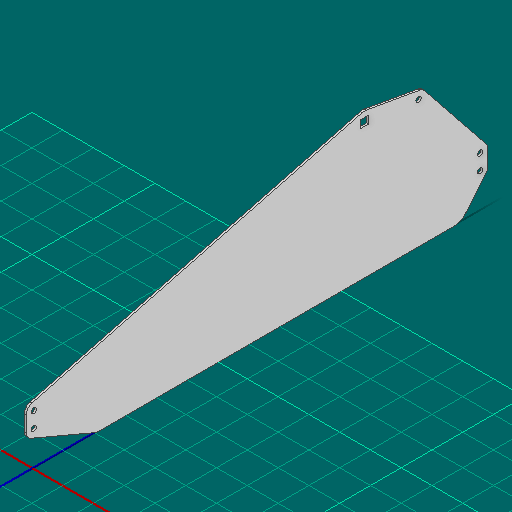
# Autodesk Inventor part: skirt_updated
Saved by Autodesk Inventor 2025 (Build 290162000, 162)
## iProperties
Created: 2024-09-29
Part Number: skirt_updated
Material: Generic
Document SubType Name: Modeling
Designer: averey
Density: 1 g/cm^3
Appearance: Default
Author: averey
Autodesk Inventor part; units mm, degrees
ref_plane "YZ Plane" through (0, 0, 0) normal (1, 0, 0) x (0, 1, 0)
ref_plane "XZ Plane" through (0, 0, 0) normal (0, 1, 0) x (-1, 0, 0)
ref_plane "XY Plane" through (0, 0, 0) normal (0, 0, 1) x (1, 0, 0)
sketch "maiin" plane through (0, 0, 0) normal (0, 0, 1) x (1, 0, 0)
  circle A0 centre (114.3234, 350.4213) radius 2.1844
  circle A1 centre (127.0234, 350.4213) radius 2.1844
  line L0 (86.4201, 300.7833) -> (108.4755, 352.8962)
  arc A2 (86.4201, 300.7833) -> (85.4157, 295.8335) centre (98.1157, 295.8335) ccw
  line L1 (209.5734, 102.7713) -> (133.0946, 352.2822)
  line L2 (209.5734, 96.4213) -> (209.5734, 102.7713)
  circle A3 centre (203.2234, 96.4213) radius 2.1844
  arc A4 (209.45, 95.176) -> (209.5734, 96.4213) centre (203.2234, 96.4213) ccw
  line L3 (196.75, 31.676) -> (209.45, 95.176)
  circle A5 centre (190.5234, 32.9213) radius 2.1844
  line L4 (85.4157, 295.8335) -> (85.4157, 3.6912)
  circle A6 centre (127.0234, -17.8787) radius 2.1844
  circle A7 centre (114.3234, -17.8787) radius 2.1844
  arc A8 (127.0234, -24.2287) -> (130.9902, -22.8372) centre (127.0234, -17.8787) ccw
  arc A9 (110.2871, -22.7809) -> (114.3234, -24.2287) centre (114.3234, -17.8787) ccw
  arc A10 (194.4902, 27.9628) -> (196.75, 31.676) centre (190.5234, 32.9213) ccw
  arc A11 (85.4157, 3.6912) -> (90.0433, -6.1132) centre (98.1157, 3.6912) ccw
  line L5 (130.9902, -22.8372) -> (194.4902, 27.9628)
  line L6 (110.2871, -22.7809) -> (90.0433, -6.1132)
  line L7 (114.3234, -24.2287) -> (127.0234, -24.2287)
  arc A12 (114.3234, 356.7713) -> (108.4755, 352.8962) centre (114.3234, 350.4213) ccw
  line L8 (127.0234, 356.7713) -> (114.3234, 356.7713)
  arc A13 (133.0946, 352.2822) -> (127.0234, 356.7713) centre (127.0234, 350.4213) ccw
  point P0 (137.6055, 139.9011)
  point P1 (110.8157, 355.7146)
  dimension "d0" = 12.7
  dimension "d1" = 12.7
  dimension "d2" = 25.4
  measures "d0" diameter of A4
  measures "d1" radius of A11
  measures "d2" distance from line of point (110.816, 355.715) L4
sketch "main" plane through (0, 0, 0) normal (0, 0, 1) x (1, 0, 0)
  line L0 (253.2515, -237.7425) -> (261.0416, -193.5682)
  circle A0 centre (170.798, 80.8603) radius 2.1844
  circle A1 centre (183.498, 80.8603) radius 2.1844
  circle A2 centre (246.998, -236.6397) radius 2.1844
  arc A3 (189.6416, 82.4661) -> (183.498, 87.2103) centre (183.498, 80.8603) ccw
  arc A4 (170.798, 87.2103) -> (164.9502, 83.3353) centre (170.798, 80.8603) ccw
  line L1 (183.498, 87.2103) -> (170.798, 87.2103)
  line L2 (141.8904, 26.2725) -> (141.8904, -265.8697)
  line L3 (260.9042, -190.1825) -> (189.6416, 82.4661)
  arc A5 (142.8948, 31.2224) -> (141.8904, 26.2725) centre (154.5904, 26.2725) ccw
  line L4 (142.8948, 31.2224) -> (164.9502, 83.3353)
  arc A6 (250.9648, -241.5982) -> (253.2515, -237.7425) centre (246.998, -236.6397) ccw
  line L5 (187.4648, -292.3982) -> (250.9648, -241.5982)
  circle A7 centre (183.498, -287.4397) radius 2.1844
  arc A8 (183.498, -293.7897) -> (187.4648, -292.3982) centre (183.498, -287.4397) ccw
  circle A9 centre (170.798, -287.4397) radius 2.1844
  line L6 (170.798, -293.7897) -> (183.498, -293.7897)
  arc A10 (166.7618, -292.3419) -> (170.798, -293.7897) centre (170.798, -287.4397) ccw
  arc A11 (141.8904, -265.8697) -> (146.518, -275.6741) centre (154.5904, -265.8697) ccw
  line L7 (166.7618, -292.3419) -> (146.518, -275.6741)
  arc A12 (261.0416, -193.5682) -> (260.9042, -190.1825) centre (253.2247, -192.1897) ccw
  point P0 (195.6606, -131.3273)
  point P1 (167.2904, 86.1536)
  dimension "d6" = 12.7
  dimension "d7" = 25.4
  dimension "d10" = 15.875
  measures "d6" radius of A11
  measures "d7" distance from line of point (167.29, 86.154) L2
  measures "d10" diameter of A12
sketch "Sketch1" plane through (0, 0, 0) normal (1, 0, 0) x (0, 1, 0)
  line L0 (73.006, -269.894) -> (66.6941, -269.894)
  line L1 (66.6941, -269.894) -> (66.6941, -276.2059)
  line L2 (66.6941, -276.2059) -> (73.006, -276.2059)
  line L3 (73.006, -276.2059) -> (73.006, -269.894)
  line L4 (73.006, -269.894) -> (66.6941, -276.2059) construction
  line L5 (66.6941, -269.894) -> (73.006, -276.2059) construction
  line L6 (69.7535, -318.6028) -> (77.5436, -274.4285)
  circle A0 centre (-12.7, 0) radius 2.1844
  circle A1 centre (0, 0) radius 2.1844
  circle A2 centre (63.5, -317.5) radius 2.1844
  arc A3 (6.1436, 1.6058) -> (0, 6.35) centre (0, 0) ccw
  arc A4 (-12.7, 6.35) -> (-18.5478, 2.4749) centre (-12.7, 0) ccw
  line L7 (0, 6.35) -> (-12.7, 6.35)
  line L8 (-41.6076, -54.5878) -> (-41.6076, -346.7301)
  line L9 (77.4062, -271.0428) -> (6.1436, 1.6058)
  arc A5 (-40.6033, -49.6379) -> (-41.6076, -54.5878) centre (-28.9076, -54.5878) ccw
  line L10 (-40.6033, -49.6379) -> (-18.5478, 2.4749)
  arc A6 (67.4668, -322.4585) -> (69.7535, -318.6028) centre (63.5, -317.5) ccw
  line L11 (3.9668, -373.2585) -> (67.4668, -322.4585)
  circle A7 centre (0, -368.3) radius 2.1844
  arc A8 (0, -374.65) -> (3.9668, -373.2585) centre (0, -368.3) ccw
  circle A9 centre (-12.7, -368.3) radius 2.1844
  line L12 (-12.7, -374.65) -> (0, -374.65)
  arc A10 (-16.7362, -373.2022) -> (-12.7, -374.65) centre (-12.7, -368.3) ccw
  arc A11 (-41.6076, -346.7301) -> (-36.98, -356.5344) centre (-28.9076, -346.7301) ccw
  line L13 (-16.7362, -373.2022) -> (-36.98, -356.5344)
  arc A12 (77.5436, -274.4285) -> (77.4062, -271.0428) centre (69.7267, -273.05) ccw
  point P0 (69.85, -273.05)
  dimension "d8" = 6.3119
  dimension "d9" = 6.3119
  constraints: 12 end point, 2 midpoint, 2 parallel, 1 horizontal, 1 perpendicular
  measures "d8" distance of L2.end L1.end
  measures "d9" distance of L1.end L0.end
extrude "Extrusion1" add sketch "Sketch1" along normal blind 1.5875
body "Solid1"
